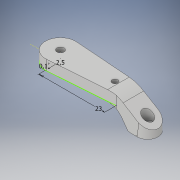
# Autodesk Inventor part: Servo-Arm-20mm-Enhanced
Saved by Autodesk Inventor 2018.2 (Build 222227000, 227)
## iProperties
Created: 2018-02-17
Part Number: Servo-Arm-20mm-Enhanced
Material: Generisch
Document SubType Name: Modeling
Designer: JochenAlt
Density: 1 g/cm^3
Appearance: Vorgabe
Author: JochenAlt
Autodesk Inventor part; units mm, degrees
ref_plane "YZ Plane" through (0, 0, 0) normal (1, 0, 0) x (0, 1, 0)
ref_plane "XZ Plane" through (0, 0, 0) normal (0, 1, 0) x (-1, 0, 0)
ref_plane "XY Plane" through (0, 0, 0) normal (0, 0, 1) x (1, 0, 0)
sketch "Skizze1" plane through (0, 0, 0) normal (0, 0, 1) x (1, 0, 0)
  line L0 (0, 5.6) -> (0, -5.6) construction
  line L1 (-9.12, 0) -> (26.72, 0) construction
  circle A0 centre (0, 0) radius 2
  circle A1 centre (9.5, 0) radius 1
  circle A2 centre (16, 0) radius 1
  circle A3 centre (19, 0) radius 1
  arc A4 (19.1916, -2.5929) -> (19.1916, 2.5929) centre (19, 0) ccw
  arc A5 (0.2947, 3.9891) -> (0.2947, -3.9891) centre (0, 0) ccw
  line L2 (0.2947, 3.9891) -> (19.1916, 2.5929)
  line L3 (0.2947, -3.9891) -> (19.1916, -2.5929)
  circle A6 centre (12.8, 0) radius 1
  circle A7 centre (0, 0) radius 4
  point P0 (0.5263, 3.9652)
  point P1 (0.6579, -1.8887)
  point P2 (0.6579, 1.8887)
  dimension "d0" = 9.5
  dimension "d1" = 16
  dimension "d2" = 19
  dimension "d3" = 5.2
  dimension "d4" = 2
  dimension "d5" = 4
  dimension "d6" = 8
  dimension "d17" = 12.8
  constraints: 7 centre point, 7 point on circle, 4 coincident, 4 end point, 4 point on line, 4 tangent, 3 equal radius, 3 other
  measures "d0" distance of A1.centre point (0, 0)
  measures "d1" distance of point (0, 0) A2.centre
  measures "d2" distance of A3.centre point (0, 0)
  measures "d3" diameter of A4
  measures "d4" diameter of A3
  measures "d5" diameter of A0
  measures "d6" diameter of A5
  measures "d17" distance of A6.centre point (0, 0)
extrude "Extrusion1" add sketch "Skizze1" along normal blind 1.8
extrude "Extrusion2" add sketch "Skizze1" against normal blind 2.7 contours A5 A7
sketch "Skizze6" plane through (0, 0, 0) normal (0, 0, 1) x (1, 0, 0)
  line L0 (0.2947, 3.9891) -> (19.1916, 2.5929) construction
  arc A0 (19.1916, -2.5929) -> (19.1916, 2.5929) centre (19, 0) ccw construction
  line L1 (19.1916, -2.5929) -> (0.2947, -3.9891) construction
  arc A1 (0.2947, 3.9891) -> (0.2947, -3.9891) centre (0, 0) ccw construction
  circle A2 centre (12.8, 0) radius 1 construction
  circle A3 centre (19, 0) radius 1 construction
  circle A4 centre (16, 0) radius 1 construction
  circle A5 centre (9.5, 0) radius 1 construction
  arc A6 (19.1989, -2.6927) -> (19.1989, 2.6927) centre (19, 0) ccw
  line L2 (19.1989, 2.6927) -> (0.3021, 4.0889)
  line L3 (23, -3.5647) -> (23, 3.5647)
  line L4 (23, 3.5647) -> (0.3868, 5.2354)
  line L5 (0.3868, -5.2354) -> (23, -3.5647)
  circle A7 centre (9.5, 0) radius 1 construction
  circle A8 centre (19, 0) radius 1
  line L6 (-10.7214, 0) -> (27.5802, 0) construction
  arc A9 (0.3868, 5.2354) -> (0.3868, -5.2354) centre (0, 0) ccw
  arc A10 (0.3021, 4.0889) -> (0.3021, -4.0889) centre (0, 0) ccw
  line L7 (0.3021, -4.0889) -> (19.1989, -2.6927)
  circle A11 centre (0, 0) radius 2 construction
  circle A12 centre (0, 0) radius 4.1
  circle A13 centre (0, 0) radius 1.25
  dimension "d106" = 2.5
  dimension "d116" = 0.1
  dimension "d117" = 23
  constraints: 10 end point, 8 centre point, 7 coincident, 6 point on circle, 6 tangent, 3 concentric, 2 parallel, 1 vertical, 1 other
  measures "d106" diameter of A13
  measures "d116" distance between parallel lines of L7 L1
  measures "d117" distance from line of L3 point (0, 0)
extrude "Extrusion11" add sketch "Skizze6" along normal blind 2 separate body contours L5 A9 L4 L3
extrude "Extrusion12" add sketch "Skizze6" along normal blind 1.5 from surface at 2 contours L7 A12 L2 A6 | A10 A12 | L5 A9 L4 L3 | A13 bodies 2
extrude "Extrusion16" cut sketch "Skizze6" along normal up to next contours A13 bodies 2
ref_plane "Arbeitsebene3" through (28, -3.5647, 0) normal (1, 0, 0) x (0, 1, 0)
ref_plane "Arbeitsebene4" through (23, -3.5647, 0) normal (1, 0, 0) x (0, 1, 0)
sketch "Skizze7" plane through (28, -3.5647, 0) normal (1, 0, 0) x (0, 1, 0)
  line L0 (7.1293, 0) -> (7.1293, 3.5) construction
  line L1 (0, 0) -> (0, 3.5) construction
  line L2 (0, 0) -> (7.1293, 0) projected
  line L3 (-0.0659, -6.75) -> (7.1952, -6.75)
  line L4 (7.1952, -6.75) -> (7.1952, -3.25)
  line L5 (7.1952, -3.25) -> (-0.0659, -3.25)
  line L6 (-0.0659, -3.25) -> (-0.0659, -6.75)
  line L7 (-0.0659, -5) -> (7.1952, -5) construction
  line L8 (3.5647, -6.75) -> (3.5647, -3.25) construction
  line L9 (3.5647, 5.55) -> (3.5647, -8.8) construction
  line L10 (7.1293, 3.5) -> (0, 3.5) projected
  point P0 (3.5647, 0)
  point P1 (3.5647, -5)
  dimension "d80" = 3.5
  dimension "d90" = 5
  constraints: 12 end point, 5 midpoint, 2 parallel, 1 perpendicular, 1 point on line
  measures "d80" distance of L4.end L3.end
  measures "d90" distance between parallel lines of L2 L7
extrude "Extrusion13" add sketch "Skizze7" along normal blind 6 bodies 2
sketch "Skizze10" plane through (28, 3.6305, -3.25) normal (0, 1, 0) x (1, 0, 0)
  line L0 (0, 3.5) -> (0, 0) construction
  line L1 (0, 0) -> (6, 0) construction
  line L2 (6, 3.5) -> (6, 0) construction
  line L3 (0, 3.5) -> (6, 3.5) construction
  line L4 (0, 3.5) -> (6, 0)
  line L5 (0, 3.5) -> (6, 3.5) construction
  line L6 (6, 3.5) -> (6, 0) construction
  line L7 (0, 3.5) -> (0, 0) projected
  line L8 (0, 3.5) -> (6, 3.5)
  line L9 (0, 0) -> (6, 0) projected
  line L10 (6, 0) -> (0, 0)
  line L11 (0, 0) -> (0, 3.5)
  point P0 (-28, -3.25)
  constraints: 8 end point, 1 collinear, 1 horizontal
extrude "Extrusion20" cut sketch "Skizze10" against normal through all bodies 2
loft "Erhebung4" add bodies 2 section 1 edges at (23, 0, 0) (23, 3.5647, 1.75) (23, 0, 3.5) (23, -3.5647, 1.75) section 2 edges at (31, -3.6305, -5) (34, 0, -3.25) (31, 3.6305, -5) (28, 0, -6.75)
fillet "Rundung2" radius 7 1 edges at (23, 0, 0)
fillet "Rundung2" radius 10 1 edges at (23, 0, 3.5)
sketch "Skizze8" plane through (24.75, -3.8379, -6.75) normal (0, 0, 1) x (1, 0, 0)
  line L0 (5.6195, 7.4684) -> (12.9438, 7.4684)
  line L1 (12.9438, 7.4684) -> (12.9438, 0.2074)
  line L2 (12.9438, 0.2074) -> (5.6195, 0.2074)
  circle A0 centre (5.6195, 3.8379) radius 3.6305
  line L3 (3.25, 7.4684) -> (9.25, 7.4684) projected
  line L4 (9.25, 0.2074) -> (9.25, 7.4684) projected
  line L5 (3.25, 0.2074) -> (9.25, 0.2074) projected
  line L6 (3.25, 0.2074) -> (9.25, 0.2074) construction
  line L7 (9.25, 0.2074) -> (9.25, 7.4684) construction
  line L8 (3.25, 7.4684) -> (9.25, 7.4684) construction
  line L9 (3.25, 0.2074) -> (3.25, 7.4684) projected
  circle A1 centre (5.6195, 3.8379) radius 0.8
  circle A2 centre (5.6195, 3.8379) radius 1.75
  point P0 (-22.2861, 3.5376)
  dimension "d114" = 1.6
  dimension "d115" = 3.5
  constraints: 6 end point, 5 tangent, 3 centre point, 3 coincident, 2 point on circle, 1 horizontal, 1 parallel, 1 perpendicular
  measures "d114" diameter of A1
  measures "d115" diameter of A2
extrude "Extrusion18" cut sketch "Skizze8" along normal through all contours L0 L4 A0 | L0 L1 L2 L4 | L4 L2 A0 | A1 bodies 2
ref_plane "Arbeitsebene5" through (30.3695, 3.6305, -3.75) normal (0, 0, -1) x (-1, 0, 0)
extrude "Extrusion19" cut sketch "Skizze8" along normal blind 5 from surface at 3 contours A1 | A2 bodies 2
chamfer "Fase5" distance 1 distance2 2 3 edges at (29.1847, -3.6305, -6.75) (34, 0, -6.75) (29.1847, 3.6305, -6.75) measured on face at (29.1847, 3.1305, -6.75) measured on face at (33.5, 0, -6.75) measured on face at (29.1847, -3.6305, -6.25)
chamfer "Fase6" distance 1 distance2 1.3 1 edges at (28, 0, -6.75) measured on face at (28.5, 0, -6.75)
fillet "Rundung4" radius 2 2 edges at (28.1514, -2.6271, -6.2502) (28.1514, 2.6271, -6.2502)
